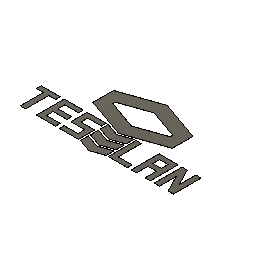
TESLAN_LOGO (Autodesk Fusion 360 design; units mm, degrees)
Autodesk Fusion 360 part; units mm, degrees
sketch "Sketch1" plane through (0, 0, 0) normal (0, 0, 1) x (1, 0, 0)
  line L0 (0, 0) -> (1149.1386, 0)
  line L1 (1149.1386, 0) -> (1149.1386, -285.624)
  line L2 (1149.1386, -285.624) -> (733.9874, -285.624)
  line L3 (733.9874, -285.624) -> (733.9874, -1673.8897)
  line L4 (733.9874, -1673.8897) -> (415.1512, -1673.8897)
  line L5 (415.1512, -1673.8897) -> (415.1512, -285.624)
  line L6 (415.1512, -285.624) -> (0, -285.624)
  line L7 (0, -285.624) -> (0, 0)
  line L8 (1149.1386, 0) -> (1381.6233, 0) construction
  line L9 (1381.6233, 0) -> (2530.7619, 0)
  line L10 (2530.7619, 0) -> (2530.7619, -285.624)
  line L11 (2530.7619, -285.624) -> (1700.4594, -285.624)
  line L12 (1700.4594, -285.624) -> (1700.4594, -694.1329)
  line L13 (1700.4594, -694.1329) -> (2530.7619, -694.1329)
  line L14 (2530.7619, -694.1329) -> (2530.7619, -979.7569)
  line L15 (2530.7619, -979.7569) -> (1700.4594, -979.7569)
  line L16 (1700.4594, -979.7569) -> (1700.4594, -1388.2657)
  line L17 (1700.4594, -1388.2657) -> (2530.7619, -1388.2657)
  line L18 (2530.7619, -1388.2657) -> (2530.7619, -1673.8897)
  line L19 (2530.7619, -1673.8897) -> (1381.6233, -1673.8897)
  line L20 (1381.6233, -1673.8897) -> (1381.6233, 0)
  line L21 (2530.7619, 0) -> (2763.2466, 0) construction
  line L22 (2763.2466, 0) -> (3912.3852, 0)
  line L23 (3912.3852, 0) -> (3912.3852, -285.624)
  line L24 (3912.3852, -285.624) -> (3082.0827, -285.624)
  line L25 (3082.0827, -285.624) -> (3082.0827, -694.1329)
  line L26 (3082.0827, -694.1329) -> (3912.3852, -694.1329)
  line L27 (3912.3852, -694.1329) -> (3912.3852, -1673.8897)
  line L28 (3912.3852, -1673.8897) -> (2763.2466, -1673.8897)
  line L29 (2763.2466, -1673.8897) -> (2763.2466, -1388.2657)
  line L30 (2763.2466, -1388.2657) -> (3593.549, -1388.2657)
  line L31 (3593.549, -1388.2657) -> (3593.549, -979.7569)
  line L32 (3593.549, -979.7569) -> (2763.2466, -979.7569)
  line L33 (2763.2466, -979.7569) -> (2763.2466, 0)
  line L34 (3912.3852, 0) -> (4031.9487, 0) construction
  line L35 (4031.9487, 0) -> (5586.2749, 0) construction
  line L36 (5586.2749, 0) -> (5705.8385, 0) construction
  line L37 (5705.8385, 0) -> (6024.6746, 0)
  line L38 (6024.6746, 0) -> (6024.6746, -1388.2657)
  line L39 (6024.6746, -1388.2657) -> (6854.977, -1388.2657)
  line L40 (6854.977, -1388.2657) -> (6854.977, -1673.8897)
  line L41 (6854.977, -1673.8897) -> (5705.8385, -1673.8897)
  line L42 (5705.8385, -1673.8897) -> (5705.8385, 0)
  line L43 (6854.977, -1388.2657) -> (7087.4617, -1388.2657) construction
  line L44 (7087.4617, -1388.2657) -> (7087.4617, 0)
  line L45 (7087.4617, 0) -> (8236.6003, 0)
  line L46 (8236.6003, 0) -> (8236.6003, -1673.8897)
  line L47 (8236.6003, -1673.8897) -> (7917.7642, -1673.8897)
  line L48 (7917.7642, -1673.8897) -> (7917.7642, -979.7569)
  line L49 (7917.7642, -979.7569) -> (7406.2979, -979.7569)
  line L50 (7406.2979, -979.7569) -> (7406.2979, -1673.8897)
  line L51 (7406.2979, -1673.8897) -> (7087.4617, -1673.8897)
  line L52 (7087.4617, -1673.8897) -> (7087.4617, -1388.2657)
  line L53 (7087.4617, 0) -> (7406.2979, 0) construction
  line L54 (7406.2979, 0) -> (7406.2979, -285.624) construction
  line L55 (7406.2979, -285.624) -> (7087.4617, -285.624) construction
  line L56 (7087.4617, -285.624) -> (7087.4617, 0) construction
  line L57 (7406.2979, -285.624) -> (7917.7642, -285.624)
  line L58 (7917.7642, -285.624) -> (7917.7642, -694.1329)
  line L59 (7917.7642, -694.1329) -> (7406.2979, -694.1329)
  line L60 (7406.2979, -694.1329) -> (7406.2979, -285.624)
  line L61 (8236.6003, 0) -> (8469.085, 0) construction
  line L62 (8469.085, 0) -> (8787.9212, 0)
  line L63 (8787.9212, 0) -> (9300.5724, -1006.1347)
  line L64 (9300.5724, -1006.1347) -> (9300.5724, 3.5131)
  line L65 (9300.5724, 3.5131) -> (9619.4085, 3.5131)
  line L66 (9619.4085, 3.5131) -> (9619.4085, -1670.3766)
  line L67 (9619.4085, -1670.3766) -> (9300.5724, -1670.3766)
  line L68 (9300.5724, -1670.3766) -> (8787.9212, -664.242)
  line L69 (8787.9212, -664.242) -> (8787.9212, -1673.8897)
  line L70 (8787.9212, -1673.8897) -> (8469.085, -1673.8897)
  line L71 (8469.085, -1673.8897) -> (8469.085, 0)
  line L72 (4031.9487, 0) -> (4031.9487, -478.2542)
  line L73 (4031.9487, -478.2542) -> (4809.2628, -750.6485)
  line L74 (4809.2628, -750.6485) -> (5586.5769, -478.2542)
  line L75 (5586.5769, -478.2542) -> (5586.5769, 0)
  line L76 (5586.5769, 0) -> (4809.2628, -272.3943)
  line L77 (4809.2628, -272.3943) -> (4031.9487, 0)
  line L78 (4031.9487, -478.2542) -> (4031.9487, -597.8178) construction
  line L79 (4031.9487, -597.8178) -> (4031.9487, -1076.072)
  line L80 (4031.9487, -1076.072) -> (4809.2628, -1348.4663)
  line L81 (4809.2628, -1348.4663) -> (5586.5769, -1076.072)
  line L82 (5586.5769, -1076.072) -> (5586.5769, -597.8178)
  line L83 (5586.5769, -597.8178) -> (4809.2628, -870.2121)
  line L84 (4809.2628, -870.2121) -> (4031.9487, -597.8178)
  line L85 (4031.9487, -1076.072) -> (4031.9487, -1195.6355) construction
  line L86 (4031.9487, -1195.6355) -> (4031.9487, -1673.8897)
  line L87 (4031.9487, -1673.8897) -> (4809.2628, -1946.284)
  line L88 (4809.2628, -1946.284) -> (5586.5769, -1673.8897)
  line L89 (5586.5769, -1673.8897) -> (5586.5769, -1195.6355)
  line L90 (5586.5769, -1195.6355) -> (4809.2628, -1468.0298)
  line L91 (4809.2628, -1468.0298) -> (4031.9487, -1195.6355)
  line L92 (4809.2628, -272.3943) -> (4809.2628, -152.8307) construction
  line L93 (4809.2628, -152.8307) -> (2418.1694, 685.0805)
  line L94 (2418.1694, 685.0805) -> (2418.1694, 1927.213)
  line L95 (2418.1694, 1927.213) -> (4809.2628, 2765.1242)
  line L96 (4809.2628, 2765.1242) -> (7200.3562, 1927.213)
  line L97 (7200.3562, 1927.213) -> (7200.3562, 685.0805)
  line L98 (7200.3562, 685.0805) -> (4809.2628, -152.8307)
  line L99 (4809.2628, 2765.1242) -> (4809.2628, 1981.3187) construction
  line L100 (4809.2628, 1981.3187) -> (3082.4658, 1376.1969)
  line L101 (3082.4658, 1376.1969) -> (3082.4658, 1222.757)
  line L102 (3082.4658, 1222.757) -> (4809.2628, 617.6353)
  line L103 (4809.2628, 617.6353) -> (6536.0598, 1222.757)
  line L104 (6536.0598, 1222.757) -> (6536.0598, 1376.1969)
  line L105 (6536.0598, 1376.1969) -> (4809.2628, 1981.3187)
  dimension "d38" = 1149.1386
  dimension "d39" = 90
  dimension "d40" = 285.624
  dimension "d41" = 90
  dimension "d42" = 415.1512
  dimension "d43" = 90
  dimension "d44" = 1388.2657
  dimension "d45" = 90
  dimension "d46" = 318.8361
  dimension "d47" = 90
  dimension "d48" = 1388.2657
  dimension "d49" = 90
  dimension "d50" = 415.1512
  dimension "d51" = 285.624
  dimension "d52" = 90
  dimension "d53" = 232.4847
  dimension "d54" = 1149.1386
  dimension "d55" = 285.624
  dimension "d56" = 90
  dimension "d57" = 830.3025
  dimension "d58" = 90
  dimension "d59" = 408.5088
  dimension "d60" = 90
  dimension "d61" = 830.3025
  dimension "d62" = 285.624
  dimension "d63" = 90
  dimension "d64" = 830.3025
  dimension "d65" = 408.5088
  dimension "d66" = 830.3025
  dimension "d67" = 285.624
  dimension "d68" = 1149.1386
  dimension "d69" = 232.4847
  dimension "d70" = 1149.1386
  dimension "d71" = 90
  dimension "d72" = 285.624
  dimension "d73" = 90
  dimension "d74" = 830.3025
  dimension "d75" = 408.5088
  dimension "d76" = 830.3025
  dimension "d77" = 979.7569
  dimension "d78" = 1149.1386
  dimension "d79" = 285.624
  dimension "d80" = 830.3025
  dimension "d81" = 408.5088
  dimension "d82" = 830.3025
  dimension "d83" = 119.5636
  dimension "d84" = 1554.3262
  dimension "d85" = 119.5636
  dimension "d86" = 318.8361
  dimension "d87" = 1388.2657
  dimension "d88" = 830.3025
  dimension "d89" = 285.624
  dimension "d90" = 1149.1386
  dimension "d91" = 1673.8897
  dimension "d92" = 232.4847
  dimension "d93" = 1388.2657
  dimension "d94" = 1149.1386
  dimension "d95" = 1673.8897
  dimension "d96" = 318.8361
  dimension "d97" = 694.1329
  dimension "d98" = 511.4663
  dimension "d99" = 694.1329
  dimension "d100" = 318.8361
  dimension "d101" = 318.8361
  dimension "d102" = 285.624
  dimension "d103" = 511.4663
  dimension "d104" = 408.5088
  dimension "d105" = 232.4847
  dimension "d106" = 318.8361
  dimension "d107" = 117
  dimension "d108" = 1129.2113
  dimension "d109" = 1009.6478
  dimension "d110" = 318.8361
  dimension "d111" = 1673.8897
  dimension "d112" = 318.8361
  dimension "d113" = 117
  dimension "d114" = 1129.2113
  dimension "d115" = 1009.6478
  dimension "d116" = 318.8361
  dimension "d117" = 478.2542
  dimension "d118" = 109.312
  dimension "d119" = 823.66
  dimension "d120" = 141.376
  dimension "d121" = 823.66
  dimension "d122" = 109.312
  dimension "d123" = 478.2542
  dimension "d124" = 70.688
  dimension "d125" = 823.66
  dimension "d126" = 119.5636
  dimension "d127" = 478.2542
  dimension "d128" = 823.66
  dimension "d129" = 109.312
  dimension "d130" = 141.376
  dimension "d131" = 823.66
  dimension "d132" = 109.312
  dimension "d133" = 478.2542
  dimension "d134" = 70.688
  dimension "d135" = 823.66
  dimension "d136" = 119.5636
  dimension "d137" = 478.2542
  dimension "d138" = 109.312
  dimension "d139" = 823.66
  dimension "d140" = 141.376
  dimension "d141" = 823.66
  dimension "d142" = 109.312
  dimension "d143" = 478.2542
  dimension "d144" = 70.688
  dimension "d145" = 823.66
  dimension "d146" = 119.5636
  dimension "d147" = 109.312
  dimension "d148" = 2533.658
  dimension "d149" = 109.312
  dimension "d150" = 1242.1325
  dimension "d151" = 109.312
  dimension "d152" = 2533.658
  dimension "d153" = 141.376
  dimension "d154" = 2533.658
  dimension "d155" = 109.312
  dimension "d156" = 1242.1325
  dimension "d157" = 783.8055
  dimension "d158" = 1829.7541
  dimension "d159" = 153.4399
  dimension "d160" = 109.312
  dimension "d161" = 109.312
  dimension "d162" = 1829.7541
  dimension "d163" = 141.376
  dimension "d164" = 1829.7541
  dimension "d165" = 109.312
  dimension "d166" = 153.4399
  constraint coincident L0.start L7.end
  constraint horizontal L0
  constraint horizontal L9
  constraint vertical L10
  constraint vertical L14
  constraint vertical L16
  constraint horizontal L17
  constraint perpendicular L4 L18
  constraint perpendicular L18 L19
  constraint horizontal L21
  constraint perpendicular L10 L22
  constraint perpendicular L9 L25
  constraint perpendicular L25 L26
  constraint perpendicular L26 L27
  constraint perpendicular L25 L28
  constraint perpendicular L28 L29
  constraint perpendicular L25 L30
  constraint perpendicular L30 L31
  constraint perpendicular L31 L32
  constraint perpendicular L23 L34
  constraint perpendicular L23 L35
  constraint perpendicular L23 L36
  constraint perpendicular L23 L37
  constraint perpendicular L34 L38
  constraint perpendicular L38 L39
  constraint perpendicular L34 L40
  constraint perpendicular L40 L41
  constraint perpendicular L37 L42
  constraint perpendicular L40 L43
  constraint perpendicular L43 L44
  constraint perpendicular L44 L45
  constraint perpendicular L43 L46
  constraint perpendicular L46 L47
  constraint perpendicular L47 L48
  constraint perpendicular L48 L49
  constraint perpendicular L47 L50
  constraint perpendicular L48 L51
  constraint horizontal L53
  constraint vertical L54
  constraint horizontal L55
  constraint vertical L56
  constraint horizontal L57
  constraint vertical L58
  constraint horizontal L59
  constraint vertical L60
  constraint perpendicular L46 L61
  constraint perpendicular L46 L62
  constraint perpendicular L45 L64
  constraint perpendicular L46 L65
  constraint perpendicular L65 L66
  constraint perpendicular L46 L67
  constraint perpendicular L65 L69
  constraint perpendicular L46 L70
  constraint perpendicular L35 L72
  constraint vertical L78
  constraint parallel L78 L79
  constraint parallel L79 L85
  constraint parallel L27 L86
  constraint perpendicular L35 L92
  constraint parallel L97 L99
  constraint parallel L95 L100
  measures "d38" distance of L0.start L0.end
  measures "d39" angle of L0 L1
  measures "d40" distance of L0.end L1.end
  measures "d41" angle of L1 L2
  measures "d42" distance of L1.end L2.end
  measures "d43" angle of L2 L3
  measures "d44" distance of L2.end L3.end
  measures "d45" angle of L3 L4
  measures "d46" distance of L3.end L4.end
  measures "d47" angle of L4 L5
  measures "d48" distance of L4.end L5.end L59
  measures "d49" angle of L5 L6
  measures "d50" distance of L5.end L6.end
  measures "d51" distance of L6.end L0.start
  measures "d52" angle of L7 L8
  measures "d53" distance of L0.end L8.end
  measures "d54" distance of L8.end L9.end
  measures "d55" distance of L9.end L10.end
  measures "d56" angle of L10 L11
  measures "d57" distance of L10.end L11.end
  measures "d58" angle of L11 L12
  measures "d59" distance of L11.end L12.end
  measures "d60" angle of L12 L13
  measures "d61" distance of L12.end L13.end
  measures "d62" distance of L13.end L14.end
  measures "d63" angle of L14 L15
  measures "d64" distance of L14.end L15.end
  measures "d65" distance of L15.end L16.end
  measures "d66" distance of L16.end L17.end
  measures "d67" distance of L17.end L18.end
  measures "d68" distance of L18.end L19.end
  measures "d69" distance of L9.end L21.end
  measures "d70" distance of L21.end L22.end
  measures "d71" angle of L22 L23
  measures "d72" distance of L22.end L23.end
  measures "d73" angle of L23 L24
  measures "d74" distance of L23.end L24.end
  measures "d75" distance of L24.end L25.end
  measures "d76" distance of L25.end L26.end
  measures "d77" distance of L26.end L27.end
  measures "d78" distance of L27.end L28.end
  measures "d79" distance of L28.end L29.end
  measures "d80" distance of L29.end L30.end
  measures "d81" distance of L30.end L31.end
  measures "d82" distance of L31.end L32.end
  measures "d83" distance of L22.end L34.end
  measures "d84" distance of L34.end L35.end
  measures "d85" distance of L35.end L36.end
  measures "d86" distance of L36.end L37.end
  measures "d87" distance of L37.end L38.end
  measures "d88" distance of L38.end L39.end
  measures "d89" distance of L39.end L40.end
  measures "d90" distance of L40.end L41.end
  measures "d91" distance of L41.end L36.end
  measures "d92" distance of L39.end L43.end
  measures "d93" distance of L43.end L44.end
  measures "d94" distance of L44.end L45.end
  measures "d95" distance of L45.end L46.end
  measures "d96" distance of L46.end L47.end
  measures "d97" distance of L47.end L48.end
  measures "d98" distance of L48.end L49.end
  measures "d99" distance of L49.end L50.end
  measures "d100" distance of L50.end L51.end
  measures "d101" distance of L44.end L53.end
  measures "d102" distance of L44.end L55.end
  measures "d103" distance of L54.end L57.end
  measures "d104" distance of L54.end L59.end
  measures "d105" distance of L45.end L61.end
  measures "d106" distance of L61.end L62.end
  measures "d107" angle of L62 L63
  measures "d108" distance of L62.end L63.end
  measures "d109" distance of L63.end L64.end
  measures "d110" distance of L64.end L65.end
  measures "d111" distance of L65.end L66.end
  measures "d112" distance of L66.end L67.end
  measures "d113" angle of L67 L68
  measures "d114" distance of L67.end L68.end
  measures "d115" distance of L68.end L69.end
  measures "d116" distance of L69.end L70.end
  measures "d117" distance of L34.end L72.end
  measures "d118" angle of L72 L73
  measures "d119" distance of L72.end L73.end
  measures "d120" angle of L73 L74
  measures "d121" distance of L73.end L74.end
  measures "d122" angle of L74 L75
  measures "d123" distance of L74.end L75.end
  measures "d124" angle of L75 L76
  measures "d125" distance of L75.end L76.end
  measures "d126" distance of L72.end L78.end
  measures "d127" distance of L78.end L79.end
  measures "d128" distance of L79.end L80.end
  measures "d129" angle of L79 L80
  measures "d130" angle of L80 L81
  measures "d131" distance of L80.end L81.end
  measures "d132" angle of L81 L82
  measures "d133" distance of L81.end L82.end
  measures "d134" angle of L82 L83
  measures "d135" distance of L82.end L83.end
  measures "d136" distance of L79.end L85.end
  measures "d137" distance of L85.end L86.end
  measures "d138" angle of L86 L87
  measures "d139" distance of L86.end L87.end
  measures "d140" angle of L87 L88
  measures "d141" distance of L87.end L88.end
  measures "d142" angle of L88 L89
  measures "d143" distance of L88.end L89.end
  measures "d144" angle of L89 L90
  measures "d145" distance of L89.end L90.end
  measures "d146" distance of L76.end L92.end
  measures "d147" angle of L92 L93
  measures "d148" distance of L92.end L93.end
  measures "d149" angle of L93 L94
  measures "d150" distance of L93.end L94.end
  measures "d151" angle of L94 L95
  measures "d152" distance of L94.end L95.end
  measures "d153" angle of L95 L96
  measures "d154" distance of L95.end L96.end
  measures "d155" angle of L96 L97
  measures "d156" distance of L96.end L97.end
  measures "d157" distance of L95.end L99.end
  measures "d158" distance of L99.end L100.end
  measures "d159" distance of L100.end L101.end
  measures "d160" angle of L100 L101
  measures "d161" angle of L101 L102
  measures "d162" distance of L101.end L102.end
  measures "d163" angle of L102 L103
  measures "d164" distance of L102.end L103.end
  measures "d165" angle of L103 L104
  measures "d166" distance of L103.end L104.end
extrude "Extrude1" add sketch "Sketch1" along normal blind 5 makes body 1 at (1487.902, -789.3409, 0) makes body 2 at (5068.3675, -500.4323, 0) makes body 3 at (521.4299, -748.3793, 0) makes body 4 at (3436.6327, 2022.8447, 0) makes body 5 at (7193.7404, -789.3409, 0) makes body 6 at (5812.1172, -1020.7185, 0) makes body 7 at (5068.3675, -1098.2501, 0) makes body 8 at (9513.1298, -890.9994, 0) makes body 9 at (5068.3675, -1696.0679, 0) makes body 10 at (2869.5253, -557.9632, 0)
equation "scaling_factor = 0.006642419620910471" comment "<-- scaling factor dimension calculator-inator"
equation "sf = scaling_factor * 1000"
equation "AA = ( 173 * sf ) * 1 mm"
equation "AB = ( 43 * sf ) * 1 mm"
equation "AC = ( 62.5 * sf ) * 1 mm"
equation "AD = ( 209 * sf ) * 1 mm"
equation "AE = ( 48 * sf ) * 1 mm"
equation "AF = ( 125 * sf ) * 1 mm"
equation "AG = ( 61.5 * sf ) * 1 mm"
equation "AH = ( 252 * sf ) * 1 mm"
equation "AI = ( 147.5 * sf ) * 1 mm"
equation "AJ = ( 72 * sf ) * 1 mm"
equation "AK = ( 124 * sf ) * 1 mm"
equation "AL = ( 104.5 * sf ) * 1 mm"
equation "AM = ( 77 * sf ) * 1 mm"
equation "AN = ( 152 * sf ) * 1 mm"
equation "AO = ( 170 * sf ) * 1 mm"
equation "AP = ( 381.436 * sf ) * 1 mm"
equation "AQ = ( 187 * sf ) * 1 mm"
equation "AR = ( 275.465 * sf ) * 1 mm"
equation "AS = ( 23.1 * sf ) * 1 mm"
equation "BA = ( 35 * sf ) * 1 mm"
equation "BB = ( 18 * sf ) * 1 mm"
equation "BC = ( 234 * sf ) * 1 mm"
equation "BD = ( 77 * sf ) * 1 mm"
equation "BE = ( 48 * sf ) * 1 mm"
equation "BF = ( 43 * sf ) * 1 mm"
equation "BH = ( 118 * sf ) * 1 mm"
equation "tw = ( 1148 * sf ) * 1 mm"
equation "th = ( 709.2 * sf ) * 1 mm"
equation "aa = 70.688 deg"
equation "ab = 109.312 deg"
equation "ac = 141.376 deg"
equation "af = 27 deg"
equation "agg = 117 deg" comment "Letop, ag was al bezet, dus deze heet agg"
equation "d38 = AA"
equation "d40 = AB"
equation "d42 = AC"
equation "d44 = AD"
equation "d46 = AE"
equation "d48 = AD"
equation "d50 = AC"
equation "d51 = AB"
equation "d53 = BA"
equation "d54 = AA"
equation "d55 = AB"
equation "d57 = AF"
equation "d59 = AG"
equation "d61 = AF"
equation "d62 = AB"
equation "d64 = AF"
equation "d65 = AG"
equation "d66 = AF"
equation "d67 = AB"
equation "d68 = AA"
equation "d69 = BA"
equation "d70 = AA"
equation "d72 = AB"
equation "d74 = AF"
equation "d75 = AG"
equation "d76 = AF"
equation "d77 = AI"
equation "d78 = AA"
equation "d79 = AB"
equation "d80 = AF"
equation "d81 = AG"
equation "d82 = AF"
equation "d83 = BB"
equation "d84 = BC"
equation "d85 = BB"
equation "d86 = AE"
equation "d87 = AD"
equation "d88 = AF"
equation "d89 = AB"
equation "d90 = AA"
equation "d91 = AH"
equation "d92 = BA"
equation "d93 = AH - AB"
equation "d94 = AA"
equation "d95 = AH"
equation "d96 = AE"
equation "d97 = AL"
equation "d98 = AM"
equation "d99 = AL"
equation "d100 = AE"
equation "d101 = BE"
equation "d102 = BF"
equation "d103 = AM"
equation "d104 = AG"
equation "d105 = BA"
equation "d106 = AE"
equation "d107 = agg"
equation "d108 = AO"
equation "d109 = AN"
equation "d110 = AE"
equation "d111 = AH"
equation "d112 = AE"
equation "d113 = agg"
equation "d114 = AO"
equation "d115 = AN"
equation "d116 = AE"
equation "d117 = AJ"
equation "d118 = ab"
equation "d119 = AK"
equation "d120 = ac"
equation "d121 = AK"
equation "d122 = ab"
equation "d123 = AJ"
equation "d124 = aa"
equation "d125 = AK"
equation "d126 = BB"
equation "d127 = AJ"
equation "d128 = AK"
equation "d129 = ab"
equation "d130 = ac"
equation "d131 = AK"
equation "d132 = ab"
equation "d133 = AJ"
equation "d134 = aa"
equation "d135 = AK"
equation "d136 = BB"
equation "d137 = AJ"
equation "d138 = ab"
equation "d139 = AK"
equation "d140 = ac"
equation "d141 = AK"
equation "d142 = ab"
equation "d143 = AJ"
equation "d144 = aa"
equation "d145 = AK"
equation "d146 = BB"
equation "d147 = 180 deg - ( ac / 2 )"
equation "d148 = AP"
equation "d149 = ab"
equation "d150 = AQ"
equation "d151 = ab"
equation "d152 = AP"
equation "d153 = ac"
equation "d154 = AP"
equation "d155 = ab"
equation "d156 = AQ"
equation "d157 = BH"
equation "d158 = AR"
equation "d159 = AS"
equation "d160 = ab"
equation "d161 = ab"
equation "d162 = AR"
equation "d163 = ac"
equation "d164 = AR"
equation "d165 = ab"
equation "d166 = AS"
